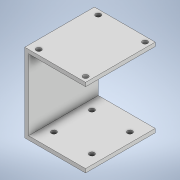
# Autodesk Inventor part: Motorhalterung_Klemme
Saved by Autodesk Inventor 2021 (Build 250183000, 183)
## iProperties
Created: 2021-01-05
Part Number: Motorhalterung_Klemme
Material: Generisch
Document SubType Name: Modeling
Designer: Ctroi
Density: 1 g/cm^3
Appearance: Vorgabe
Author: Ctroi
Autodesk Inventor part; units mm, degrees
ref_plane "YZ Plane" through (0, 0, 0) normal (1, 0, 0) x (0, 1, 0)
ref_plane "XZ Plane" through (0, 0, 0) normal (0, 1, 0) x (-1, 0, 0)
ref_plane "XY Plane" through (0, 0, 0) normal (0, 0, 1) x (1, 0, 0)
sketch "Skizze2" plane through (0, 0, 0) normal (1, 0, 0) x (0, 1, 0)
  line L0 (-43.4, 0) -> (43.4, 0) projected
  line L1 (0, -38.5) -> (0, 38.5) projected
  line L2 (31, 27.5) -> (-31, 27.5)
  line L3 (-31, 27.5) -> (-31, -27.5)
  line L4 (-31, -27.5) -> (31, -27.5)
  line L5 (31, -27.5) -> (31, 27.5)
  dimension "d5" = 62
  dimension "d6" = 55
  constraints: 8 end point, 2 parallel, 1 horizontal, 1 perpendicular, 2 other
  measures "d5" distance of L4.end L3.end
  measures "d6" distance of L3.end L2.end
extrude "Extrusion1" add sketch "Skizze2" along normal blind 3
sketch "Skizze3" plane through (3, 0, 0) normal (1, 0, 0) x (0, 0, -1)
  line L0 (-27.5, 31) -> (-27.5, -31) projected
  line L1 (27.5, -31) -> (27.5, 31) projected
  line L2 (-27.5, -31) -> (27.5, -31)
  line L3 (27.5, -31) -> (27.5, -28)
  line L4 (27.5, -28) -> (-27.5, -28)
  line L5 (-27.5, -28) -> (-27.5, -31)
  line L6 (27.5, 31) -> (-27.5, 31) projected
  line L7 (-27.5, 31) -> (27.5, 31)
  line L8 (27.5, 31) -> (27.5, 28)
  line L9 (27.5, 28) -> (-27.5, 28)
  line L10 (-27.5, 28) -> (-27.5, 31)
  point P0 (0, 0)
  dimension "d9" = 3
  dimension "d10" = 3
  constraints: 16 end point, 4 parallel, 2 horizontal, 2 perpendicular, 2 point on line
  measures "d9" distance of L3.end L2.end
  measures "d10" distance of L7.end L8.end
extrude "Extrusion2" add sketch "Skizze3" along normal blind 45 contours L6 L1 L9 L0 | L4 L1 L2 L0
sketch "Skizze5" plane through (0, 31, 27.5) normal (0, 1, 0) x (1, 0, 0)
  line L0 (0, 55) -> (0, 0) projected
  line L1 (0, 0) -> (48, 0) projected
  line L2 (0, 55) -> (48, 55) projected
  line L3 (48, 55) -> (48, 0) projected
  circle A0 centre (7, 4) radius 2
  circle A1 centre (7, 51) radius 2
  circle A2 centre (44, 51) radius 2
  circle A3 centre (44, 4) radius 2
  point P0 (0, 27.5)
  dimension "d38" = 4
  dimension "d41" = 4
  dimension "d44" = 4
  dimension "d47" = 4
  dimension "d69" = 7
  dimension "d70" = 4
  dimension "d71" = 4
  dimension "d72" = 7
  dimension "d73" = 4
  dimension "d74" = 4
  dimension "d75" = 4
  dimension "d76" = 4
  constraints: 4 centre point
  measures "d38" diameter of A0
  measures "d41" diameter of A1
  measures "d44" diameter of A2
  measures "d47" diameter of A3
  measures "d69" distance from line of L0 A1.centre
  measures "d70" distance from line of L2 A1.centre
  measures "d71" distance from line of L1 A0.centre
  measures "d72" distance from line of L0 A0.centre
  measures "d73" distance from line of L3 A3.centre
  measures "d74" distance from line of L1 A3.centre
  measures "d75" distance from line of L3 A2.centre
  measures "d76" distance from line of L2 A2.centre
extrude "Extrusion3" cut sketch "Skizze5" against normal up to surface (3 mm away) contours A0 | A1 | A2 | A3
sketch "Skizze6" plane through (0, -31, -27.5) normal (0, -1, 0) x (1, 0, 0)
  circle A0 centre (40.5, 42.5) radius 2
  circle A1 centre (40.5, 12.5) radius 2
  line L0 (0, 0) -> (48, 0) projected
  line L1 (48, 55) -> (48, 0) projected
  circle A2 centre (10.5, 42.5) radius 2
  circle A3 centre (10.5, 12.5) radius 2
  line L2 (0, 0) -> (0, 55) projected
  point P0 (0, 27.5)
  dimension "d52" = 4
  dimension "d53" = 4
  dimension "d59" = 12.5
  dimension "d62" = 7.5
  dimension "d63" = 4
  dimension "d65" = 4
  dimension "d78" = 10.5
  constraints: 4 centre point
  measures "d52" diameter of A0
  measures "d53" diameter of A1
  measures "d59" distance from line of L0 A1.centre
  measures "d62" distance from line of L1 A0.centre
  measures "d63" diameter of A2
  measures "d65" diameter of A3
  measures "d78" distance from line of L2 A3.centre
extrude "Extrusion4" cut sketch "Skizze6" against normal up to surface (3 mm away)
